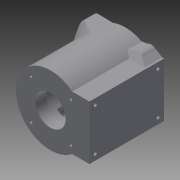
# Autodesk Inventor part: motorSupport-ExFlex-Part2
Saved by Autodesk Inventor 2014 SP2 (Build 180246200, 246)
## iProperties
Created: 2020-04-11
Part Number: motorSupport-ExFlex-Part2
Material: Generic
Document SubType Name: Sheet Metal
Designer: GauchoHP
Density: 1 g/cm^3
Sheet Metal Rule: Default_mm
Appearance: Default
Author: GauchoHP
Autodesk Inventor part; units mm, degrees
ref_plane "YZ Plane" through (0, 0, 0) normal (1, 0, 0) x (0, 1, 0)
ref_plane "XZ Plane" through (0, 0, 0) normal (0, 1, 0) x (-1, 0, 0)
ref_plane "XY Plane" through (0, 0, 0) normal (0, 0, 1) x (1, 0, 0)
sketch "Sketch1" plane through (0, 0, 0) normal (0, 1, 0) x (-1, 0, 0)
  circle A0 centre (0, 0) radius 14
  circle A1 centre (0, 0) radius 32
  line L0 (-18.3848, -18.3848) -> (18.3848, 18.3848)
  line L1 (-18.3848, 18.3848) -> (18.3848, -18.3848)
  circle A2 centre (-18.3848, 18.3848) radius 1.5
  circle A3 centre (18.3848, 18.3848) radius 1.5
  circle A4 centre (-18.3848, -18.3848) radius 1.5
  circle A5 centre (18.3848, -18.3848) radius 1.5
  arc A6 (17.294, 19.4144) -> (-17.294, 19.4144) centre (0, 0) ccw
  arc A7 (19.4144, -17.294) -> (19.4144, 17.294) centre (0, 0) ccw
  arc A8 (-19.4144, 17.294) -> (-19.4144, -17.294) centre (0, 0) ccw
  arc A9 (-17.294, -19.4144) -> (17.294, -19.4144) centre (0, 0) ccw
  dimension "d0" = 28
  dimension "d2" = 64
  dimension "d3" = 3
  dimension "d4" = 3
  dimension "d5" = 3
  dimension "d6" = 3
  constraints: 16 point on circle, 10 centre point, 7 coincident, 4 end point
  measures "d0" diameter of A0
  measures "d2" diameter of A1
  measures "d3" diameter of A2
  measures "d4" diameter of A3
  measures "d5" diameter of A4
  measures "d6" diameter of A5
extrude "Extrusion1" add sketch "Sketch1" along normal blind 10 contours A0 L0 A3 A7 A5 L1 | A0 L1 A2 A6 A3 L0 | L1 A5 A9 A4 L0 A0 | A0 L0 A4 A8 A2 L1 | A1
sketch "Sketch2" plane through (0, 10, 0) normal (0, 1, 0) x (1, 0, 0)
  circle A0 centre (18.3848, 18.3848) radius 1.5 projected
  circle A1 centre (-18.3848, 18.3848) radius 1.5 projected
  circle A2 centre (-18.3848, -18.3848) radius 1.5 projected
  circle A3 centre (18.3848, -18.3848) radius 1.5 projected
  circle A4 centre (0, 0) radius 32 projected
  circle A5 centre (0, 0) radius 18.5
  dimension "d9" = 37
  constraints: 1 centre point, 1 coincident
  measures "d9" diameter of A5
extrude "Extrusion2" add sketch "Sketch2" along normal blind 59
sketch "Sketch3" plane through (0, 69, 0) normal (0, 1, 0) x (1, 0, 0)
  circle A0 centre (0, 0) radius 18.5 projected
  circle A1 centre (-18.3848, -18.3848) radius 1.5 projected
  circle A2 centre (0, 0) radius 32 projected
  line L0 (15, -20) -> (15, -14)
  line L1 (-15, -14) -> (-15, -20)
  line L2 (-14.9373, -21) -> (-15, -21)
  line L3 (-15, -21) -> (-15, -14)
  line L4 (14.9373, -21) -> (15, -21)
  line L5 (15, -21) -> (15, -14)
  arc A3 (-15, -20) -> (-13.6497, -24.4476) centre (-7, -20) ccw
  arc A4 (13.6497, -24.4476) -> (15, -20) centre (7, -20) ccw
  arc A5 (-13.6497, -24.4476) -> (13.6497, -24.4476) centre (0, 0) ccw
  line L6 (0, -28) -> (0, -25.5017)
  circle A6 centre (18.3848, -18.3848) radius 1.5 projected
  line L7 (-17.6693, 0) -> (17.6693, 0)
  line L8 (-15, -14) -> (15, -14)
  circle A7 centre (-18.3848, 18.3848) radius 1.5
  line L9 (15, 20) -> (15, 14)
  line L10 (-15, 14) -> (-15, 20)
  line L11 (-14.9373, 21) -> (-15, 21)
  line L12 (-15, 21) -> (-15, 14)
  line L13 (14.9373, 21) -> (15, 21)
  line L14 (15, 21) -> (15, 14)
  arc A8 (-13.6497, 24.4476) -> (-15, 20) centre (-7, 20) ccw
  arc A9 (15, 20) -> (13.6497, 24.4476) centre (7, 20) ccw
  arc A10 (13.6497, 24.4476) -> (-13.6497, 24.4476) centre (0, 0) ccw
  line L15 (0, 28) -> (0, 25.5017)
  circle A11 centre (18.3848, 18.3848) radius 1.5
  line L16 (-15, 14) -> (15, 14)
  point P0 (15, -28)
  point P1 (-20.8494, -14)
  point P2 (11.2895, -14.656)
  point P3 (15, 28)
  point P4 (-20.8494, 14)
  point P5 (11.2895, 14.656)
  dimension "d12" = 30
  dimension "d13" = 14
  dimension "d14" = 15
  dimension "d22" = 8
  dimension "d26" = 28
  dimension "d27" = 8
  dimension "d28" = 30
  dimension "d29" = 3.3848
  dimension "d35" = 15
  dimension "d38" = 14
  dimension "d39" = 14
  dimension "d40" = 0
  constraints: 34 end point, 19 symmetric about line, 17 point on circle, 8 centre point, 2 point on line, 2 tangent, 1 equal radius, 1 parallel, 1 perpendicular, 7 other
  measures "d12" distance of L1.start L0.end
  measures "d13" distance of L0.end point (15, -28)
  measures "d14" distance from line of L1 point (0, 0)
  measures "d22" radius of A3
  measures "d26" radius of A5
  measures "d27" radius of A4
  measures "d28" distance between parallel lines of L0 L1
  measures "d29" distance from line of A1.centre L1
  measures "d35" distance from line of A2.centre L1
  measures "d38" distance between parallel lines of L7 L8
  measures "d39" distance from line of L6.start L8
  measures "d40" distance from line of L7 A2.centre
extrude "Extrusion3" cut sketch "Sketch3" against normal blind 51 contours L16 A0 | A0 L16 L10 A8 A10 A9 L9 | L8 L0 A4 A5 A3 L1 A0 | A0 L8
sketch "Sketch5" plane through (0, 69, 0) normal (0, 1, 0) x (1, 0, 0)
  circle A0 centre (0, 0) radius 32 projected
  line L0 (19.975, -25) -> (36, -25)
  line L1 (36, -25) -> (36, 25)
  line L2 (36, 25) -> (19.975, 25)
  line L3 (15.6974, 25) -> (15.6974, -25)
  dimension "d41" = 36
  dimension "d42" = 50
  dimension "d43" = 25
  constraints: 8 end point, 2 parallel, 2 point on circle, 1 horizontal, 1 perpendicular
  measures "d41" distance from line of L1 A0.centre
  measures "d42" distance between parallel lines of L0 L2
  measures "d43" distance from line of L2 A0.centre
extrude "Extrusion4" add sketch "Sketch5" against normal blind 69 contours A0 L2 L1 L0
sketch "Sketch6" plane through (36, 69, 25) normal (1, 0, 0) x (0, 0, -1)
  line L0 (0, 0) -> (50, 0) projected
  line L1 (0, 0) -> (0, -69) projected
  line L2 (50, -69) -> (0, -69) projected
  line L3 (50, 0) -> (50, -69) projected
  line L4 (5.5, -5.5) -> (44.5, -5.5)
  line L5 (44.5, -5.5) -> (44.5, -63.5)
  line L6 (44.5, -63.5) -> (5.5, -63.5)
  line L7 (5.5, -63.5) -> (5.5, -5.5)
  circle A0 centre (5.5, -5.5) radius 1.5
  circle A1 centre (44.5, -5.5) radius 1.5
  circle A2 centre (44.5, -63.5) radius 1.5
  circle A3 centre (5.5, -63.5) radius 1.5
  point P0 (25, -69)
  dimension "d46" = 5.5
  dimension "d47" = 5.5
  dimension "d48" = 5.5
  dimension "d49" = 5.5
  dimension "d50" = 3
  dimension "d51" = 3
  dimension "d52" = 3
  dimension "d53" = 3
  constraints: 8 end point, 4 centre point, 4 coincident, 2 parallel, 1 horizontal, 1 perpendicular
  measures "d46" distance between parallel lines of L1 L7
  measures "d47" distance between parallel lines of L3 L5
  measures "d48" distance between parallel lines of L0 L4
  measures "d49" distance between parallel lines of L6 L2
  measures "d50" diameter of A0
  measures "d51" diameter of A1
  measures "d52" diameter of A2
  measures "d53" diameter of A3
extrude "Extrusion5" cut sketch "Sketch6" against normal blind 12 contours L7 A0 L4 | L4 A0 L7 | A1 L5 L4 | L4 L5 A1 | A3 L6 L7 | L7 L6 A3 | A2 L6 L5 | L5 L6 A2
sketch "Sketch7" plane through (0, 69, 0) normal (0, 1, 0) x (1, 0, 0)
  arc A0 (19.975, 25) -> (19.975, -25) centre (0, 0) ccw projected
  line L0 (-24.25, 24.25) -> (24.25, 24.25)
  line L1 (24.25, 24.25) -> (24.25, -24.25)
  line L2 (24.25, -24.25) -> (-24.25, -24.25)
  line L3 (-24.25, -24.25) -> (-24.25, 24.25)
  circle A1 centre (-24.25, 24.25) radius 2
  circle A2 centre (24.25, 24.25) radius 2
  circle A3 centre (24.25, -24.25) radius 2
  circle A4 centre (-24.25, -24.25) radius 2
  circle A5 centre (-24.25, 24.25) radius 6
  circle A6 centre (24.25, 24.25) radius 6
  circle A7 centre (24.25, -24.25) radius 6
  circle A8 centre (-24.25, -24.25) radius 6
  dimension "d56" = 48.5
  dimension "d57" = 48.5
  dimension "d58" = 24.25
  dimension "d59" = 24.25
  dimension "d60" = 4
  dimension "d61" = 4
  dimension "d62" = 4
  dimension "d63" = 4
  dimension "d64" = 12
  dimension "d65" = 12
  dimension "d66" = 12
  dimension "d67" = 12
  constraints: 8 centre point, 8 coincident, 8 end point, 2 parallel, 1 horizontal, 1 perpendicular
  measures "d56" distance of L1.end L2.end
  measures "d57" distance of L0.end L1.end
  measures "d58" distance from line of L3 A0.centre
  measures "d59" distance from line of L0 A0.centre
  measures "d60" diameter of A1
  measures "d61" diameter of A2
  measures "d62" diameter of A3
  measures "d63" diameter of A4
  measures "d64" diameter of A5
  measures "d65" diameter of A6
  measures "d66" diameter of A7
  measures "d67" diameter of A8
extrude "Extrusion6" add sketch "Sketch7" against normal blind 10 contours A6 L1 A2 L0 | A5 L0 A0 | A0 L0 A1 L3 A5 | L0 A2 L1 A6 | L0 A5 L3 A0 | A0 L3 A1 L0 | A0 L3 A5 | A8 L3 A0 | A0 L3 A4 L2 A8 | A7 L2 A3 L1 | L1 A3 L2 A7 | A8 L2 A0 L3 | A0 L2 A4 L3 | A0 L2 A8
sketch "Sketch8" plane through (0, 59, 0) normal (0, -1, 0) x (1, 0, 0)
  arc A0 (-26.084, -18.5372) -> (-18.5372, -26.084) centre (0, 0) ccw projected
  arc A1 (-26.084, -18.5372) -> (-18.5372, -26.084) centre (-24.25, -24.25) ccw projected
extrude "Extrusion7" add sketch "Sketch8" along normal blind 1
sketch "Sketch9" plane through (0, 59, 0) normal (0, -1, 0) x (1, 0, 0)
  arc A0 (-18.5372, 26.084) -> (-26.084, 18.5372) centre (0, 0) ccw projected
  arc A1 (-18.5372, 26.084) -> (-26.084, 18.5372) centre (-24.25, 24.25) ccw projected
extrude "Extrusion8" add sketch "Sketch9" along normal blind 1
sketch "Sketch10" plane through (0, 59, 0) normal (0, -1, 0) x (1, 0, 0)
  line L0 (19.975, -25) -> (22.396, -25) projected
  arc A0 (18.5372, -26.084) -> (19.975, -25) centre (0, 0) ccw projected
  arc A1 (18.5372, -26.084) -> (30.2029, -25) centre (24.25, -24.25) ccw projected
  line L1 (26.104, -25) -> (30.2029, -25) projected
  arc A2 (22.396, -25) -> (26.104, -25) centre (24.25, -24.25) ccw projected
  line L2 (22.396, -25) -> (26.104, -25)
  constraints: 2 end point, 1 collinear
extrude "Extrusion9" add sketch "Sketch10" along normal blind 1
sketch "Sketch11" plane through (0, 59, 0) normal (0, -1, 0) x (1, 0, 0)
  line L0 (22.396, 25) -> (19.975, 25) projected
  arc A0 (26.104, 25) -> (22.396, 25) centre (24.25, 24.25) ccw projected
  line L1 (30.2029, 25) -> (26.104, 25) projected
  arc A1 (30.2029, 25) -> (18.5372, 26.084) centre (24.25, 24.25) ccw projected
  arc A2 (19.975, 25) -> (18.5372, 26.084) centre (0, 0) ccw projected
  line L2 (22.396, 25) -> (26.104, 25)
  constraints: 2 end point, 1 collinear
extrude "Extrusion10" add sketch "Sketch11" along normal blind 1
chamfer "Chamfer1" distance 5.24 angle 45 1 edges at (25.089, 58, 25)
chamfer "Chamfer2" distance 5.24 angle 45 1 edges at (25.089, 58, -25)
chamfer "Chamfer3" distance 8.29 angle 45 1 edges at (-22.6274, 58, -22.6274)
chamfer "Chamfer4" distance 8.29 angle 45 1 edges at (-22.6274, 58, 22.6274)
sketch "Sketch12" plane through (0, 69, 0) normal (0, 1, 0) x (1, 0, 0)
  line L0 (26.104, 25) -> (22.396, 25) projected
  arc A0 (26.104, 25) -> (22.396, 25) centre (24.25, 24.25) ccw projected
  line L1 (22.396, -25) -> (26.104, -25) projected
  arc A1 (22.396, -25) -> (26.104, -25) centre (24.25, -24.25) ccw projected
  arc A2 (30.2029, 25) -> (18.5372, 26.084) centre (24.25, 24.25) ccw projected
  arc A3 (18.5372, -26.084) -> (30.2029, -25) centre (24.25, -24.25) ccw projected
  circle A4 centre (24.25, 24.25) radius 2
  circle A5 centre (24.25, -24.25) radius 2
  constraints: 2 coincident, 6 other
extrude "Extrusion11" cut sketch "Sketch12" against normal blind 10 contours A4 L0 | A5 L1
chamfer "Chamfer5" distance 8 angle 45 12 edges at (-18.5372, 53.855, -26.084) (-18.5372, 58.5, -26.084) (-18.5372, 64, -26.084) (-26.084, 64, -18.5372) (-26.084, 58.5, -18.5372) (-26.084, 53.855, -18.5372) (-26.084, 53.855, 18.5372) (-26.084, 58.5, 18.5372) (-26.084, 64, 18.5372) (-18.5372, 53.855, 26.084) (-18.5372, 58.5, 26.084) (-18.5372, 64, 26.084)
chamfer "Chamfer6" distance 4 angle 45 8 edges at (18.5372, 64, -26.084) (18.5372, 56.422, -26.084) (30.2029, 64, -25) (30.2029, 55.88, -25) (30.2029, 64, 25) (30.2029, 55.88, 25) (18.5372, 64, 26.084) (18.5372, 56.422, 26.084)
sketch "Sketch13" plane through (0, 69, 0) normal (0, 1, 0) x (1, 0, 0)
  circle A0 centre (18.3848, -18.3848) radius 1.5 projected
  circle A1 centre (-18.3848, -18.3848) radius 1.5 projected
  circle A2 centre (-18.3848, 18.3848) radius 1.5 projected
  circle A3 centre (18.3848, 18.3848) radius 1.5 projected
extrude "Extrusion12" add sketch "Sketch13" against normal blind 50
equation "\"BendRadius\" = Thickness"
equation "\"BendReliefWidth\" = Thickness"
equation "\"BendReliefDepth\" = 0.5 * Thickness"
equation "\"CornerReliefSize\" = 4 * Thickness"
equation "\"MinimumRemnant\" = 2 * Thickness"
equation "\"TransitionRadius\" = BendRadius"
equation "\"JacobiRadiusSize\" = BendRadius"
equation "\"GapSize\" = Thickness"
equation "\"Thickness\" = 0.5"
body "Solid1"
